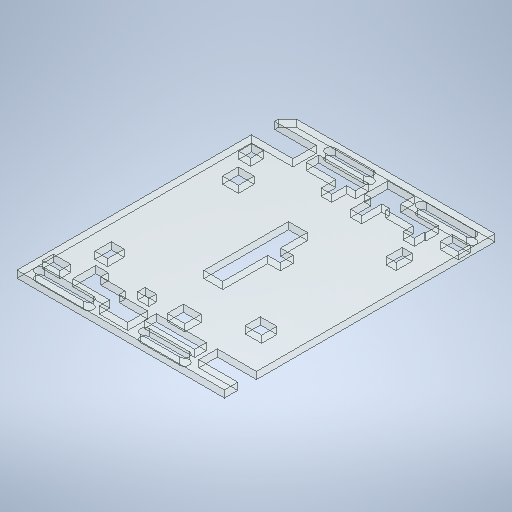
# Autodesk Inventor part: Flex Holder V1
Saved by Autodesk Inventor 2025 (Build 290162000, 162)
## iProperties
Created: 2025-07-01
Part Number: Flex Holder V1
Material: Thermoplastic Resin
Document SubType Name: Modeling
Designer: Caleb Fangmeier
Density: 1.28 g/cm^3
Appearance: Clear
Author: Caleb Fangmeier
Autodesk Inventor part; units mm, degrees
ref_plane "YZ Plane" through (0, 0, 0) normal (1, 0, 0) x (0, 1, 0)
ref_plane "XZ Plane" through (0, 0, 0) normal (0, 1, 0) x (-1, 0, 0)
ref_plane "XY Plane" through (0, 0, 0) normal (0, 0, 1) x (1, 0, 0)
sketch "Sketch1" plane through (0, 0, 0) normal (0, 1, 0) x (-1, 0, 0)
  line L0 (-22.05, -28.75) -> (22.05, -28.75)
  line L1 (22.05, -28.75) -> (22.05, 28.75)
  line L2 (22.05, 28.75) -> (-22.05, 28.75)
  line L3 (-22.05, 28.75) -> (-22.05, -28.75)
  line L4 (-22.05, -28.75) -> (22.05, 28.75) construction
  line L5 (22.05, -28.75) -> (-22.05, 28.75) construction
  point P0 (0, 0)
  dimension "d0" = 57.5
  dimension "d1" = 44.1
  constraints: 12 end point, 2 midpoint, 2 parallel, 1 horizontal, 1 perpendicular
  measures "d0" distance of L0.end L1.end
  measures "d1" distance of L1.end L2.end
extrude "Extrusion1" add sketch "Sketch1" along normal blind 1.5
sketch "Sketch4" plane through (0, 1.5, 0) normal (0, 1, 0) x (1, 0, 0)
  line L0 (22.6381, -25.9185) -> (13.7388, -25.9185)
  line L1 (13.7388, -25.9185) -> (13.7388, -21.956)
  line L2 (13.7388, -21.956) -> (22.6381, -21.956)
  line L3 (22.6381, -21.956) -> (22.6381, -25.9185)
  line L4 (11.4165, -21.956) -> (0.7633, -21.956)
  line L5 (0.7633, -21.956) -> (0.7633, -24.4569)
  line L6 (0.7633, -24.4569) -> (11.4165, -24.4569)
  line L7 (11.4165, -24.4569) -> (11.4165, -21.956)
  line L8 (-0.6658, -26.6006) -> (-6.707, -26.6006)
  line L9 (-6.707, -26.6006) -> (-6.707, -22.3783)
  line L10 (-6.707, -22.3783) -> (-0.6658, -22.3783)
  line L11 (-0.6658, -22.3783) -> (-0.6658, -26.6006)
  line L12 (-6.707, -24.392) -> (-14.5426, -24.392)
  line L13 (-14.5426, -24.392) -> (-14.5426, -21.0953)
  line L14 (-14.5426, -21.0953) -> (-6.707, -21.0953)
  line L15 (-6.707, -21.0953) -> (-6.707, -24.392)
  line L16 (-14.5426, -21.0953) -> (-11.8996, -21.0953)
  line L17 (-11.8996, -21.0953) -> (-11.8996, -19.5363)
  line L18 (-11.8996, -19.5363) -> (-14.5426, -19.5363)
  line L19 (-14.5426, -19.5363) -> (-14.5426, -21.0953)
  line L20 (-21.1238, -24.2621) -> (-17.4211, -24.2621)
  line L21 (-17.4211, -24.2621) -> (-17.4211, -21.956)
  line L22 (-17.4211, -21.956) -> (-21.1238, -21.956)
  line L23 (-21.1238, -21.956) -> (-21.1238, -24.2621)
  line L24 (5.6616, -20.7705) -> (1.894, -20.7705)
  line L25 (1.894, -20.7705) -> (1.894, -17.3277)
  line L26 (1.894, -17.3277) -> (5.6616, -17.3277)
  line L27 (5.6616, -17.3277) -> (5.6616, -20.7705)
  line L28 (-2.848, -19.9261) -> (-5.2515, -19.9261)
  line L29 (-5.2515, -19.9261) -> (-5.2515, -18.3346)
  line L30 (-5.2515, -18.3346) -> (-2.848, -18.3346)
  line L31 (-2.848, -18.3346) -> (-2.848, -19.9261)
  line L32 (-17.2689, -17.0029) -> (-14.5426, -17.0029)
  line L33 (-14.5426, -17.0029) -> (-14.5426, -13.4952)
  line L34 (-14.5426, -13.4952) -> (-17.2689, -13.4952)
  line L35 (-17.2689, -13.4952) -> (-17.2689, -17.0029)
  line L36 (15.925, -11.4814) -> (12.4173, -11.4814)
  line L37 (12.4173, -11.4814) -> (12.4173, -14.7294)
  line L38 (12.4173, -14.7294) -> (15.925, -14.7294)
  line L39 (15.925, -14.7294) -> (15.925, -11.4814)
  line L40 (-2.1335, 9.0455) -> (1.894, 9.0455)
  line L41 (1.894, 9.0455) -> (1.894, -8.9481)
  line L42 (1.894, -8.9481) -> (-2.1335, -8.9481)
  line L43 (-2.1335, -8.9481) -> (-2.1335, 9.0455)
  line L44 (4.5573, 3.3291) -> (1.6991, 3.3291)
  line L45 (1.6991, 3.3291) -> (1.6991, 0.6009)
  line L46 (1.6991, 0.6009) -> (4.5573, 0.6009)
  line L47 (4.5573, 0.6009) -> (4.5573, 3.3291)
  line L48 (-17.5287, 13.7631) -> (-14.1519, 13.7631)
  line L49 (-14.1519, 13.7631) -> (-14.1519, 10.4096)
  line L50 (-14.1519, 10.4096) -> (-17.5287, 10.4096)
  line L51 (-17.5287, 10.4096) -> (-17.5287, 13.7631)
  line L52 (16.8052, 16.3739) -> (14.7212, 16.3739)
  line L53 (14.7212, 16.3739) -> (14.7212, 12.9633)
  line L54 (14.7212, 12.9633) -> (16.8052, 12.9633)
  line L55 (16.8052, 12.9633) -> (16.8052, 16.3739)
  line L56 (-23.3919, 26.0219) -> (-13.2211, 26.0219)
  line L57 (-13.2211, 26.0219) -> (-13.2211, 21.0711)
  line L58 (-13.2211, 21.0711) -> (-23.3919, 21.0711)
  line L59 (-23.3919, 21.0711) -> (-23.3919, 26.0219)
  line L60 (-20.3793, 16.7032) -> (-17.8455, 16.7032)
  line L61 (-17.8455, 16.7032) -> (-17.8455, 19.4346)
  line L62 (-17.8455, 19.4346) -> (-20.3793, 19.4346)
  line L63 (-20.3793, 19.4346) -> (-20.3793, 16.7032)
  line L64 (-11.1745, 21.8169) -> (-0.7032, 21.8169)
  line L65 (-0.7032, 21.8169) -> (-0.7032, 24.5446)
  line L66 (-0.7032, 24.5446) -> (-11.1745, 24.5446)
  line L67 (-11.1745, 24.5446) -> (-11.1745, 21.8169)
  line L68 (-2.5673, 18.6812) -> (-4.8458, 18.6812)
  line L69 (-4.8458, 18.6812) -> (-4.8458, 22.2038)
  line L70 (-4.8458, 22.2038) -> (-2.5673, 22.2038)
  line L71 (-2.5673, 22.2038) -> (-2.5673, 18.6812)
  line L72 (0.9146, 27.1153) -> (6.539, 27.1153)
  line L73 (6.539, 27.1153) -> (6.539, 22.2038)
  line L74 (6.539, 22.2038) -> (0.9146, 22.2038)
  line L75 (0.9146, 22.2038) -> (0.9146, 27.1153)
  line L76 (2.2307, 17.9158) -> (4.5573, 17.9158)
  line L77 (4.5573, 17.9158) -> (4.5573, 22.2038)
  line L78 (4.5573, 22.2038) -> (2.2307, 22.2038)
  line L79 (2.2307, 22.2038) -> (2.2307, 17.9158)
  line L80 (6.0899, 24.1958) -> (14.5454, 24.1958)
  line L81 (14.5454, 24.1958) -> (14.5454, 21.5323)
  line L82 (14.5454, 21.5323) -> (6.0899, 21.5323)
  line L83 (6.0899, 21.5323) -> (6.0899, 24.1958)
  line L84 (14.2886, 21.5323) -> (11.9019, 21.5323)
  line L85 (11.9019, 21.5323) -> (11.9019, 19.3557)
  line L86 (11.9019, 19.3557) -> (14.2886, 19.3557)
  line L87 (14.2886, 19.3557) -> (14.2886, 21.5323)
  line L88 (21.4363, 24.0758) -> (17.64, 24.0758)
  line L89 (17.64, 24.0758) -> (17.64, 21.5323)
  line L90 (17.64, 21.5323) -> (21.4363, 21.5323)
  line L91 (21.4363, 21.5323) -> (21.4363, 24.0758)
  point P0 (0, 0)
  point P1 (6.539, 24.1958)
  point P2 (6.0899, 22.2038)
  constraints: 184 end point, 46 parallel, 23 perpendicular, 22 horizontal, 3 point on line
extrude "Clearance Cutouts" cut sketch "Sketch4" against normal blind 1.5
sketch "Sketch5" plane through (0, 1.5, 0) normal (0, 1, 0) x (1, 0, 0)
  line L0 (19.55, 26.1958) -> (9.039, 26.1958) construction
  line L1 (19.55, 27.1958) -> (9.039, 27.1958)
  line L2 (9.039, 25.1958) -> (19.55, 25.1958)
  arc A0 (19.55, 25.1958) -> (19.55, 27.1958) centre (19.55, 26.1958) ccw
  arc A1 (9.039, 27.1958) -> (9.039, 25.1958) centre (9.039, 26.1958) ccw
  line L3 (6.539, 24.1958) -> (14.5454, 24.1958) projected
  line L4 (6.539, 27.1153) -> (6.539, 24.1958) projected
  line L5 (22.05, -21.956) -> (22.05, 28.75) projected
  line L6 (-2.5854, 26.5446) -> (-10.7211, 26.5446) construction
  line L7 (-2.5854, 25.5446) -> (-10.7211, 25.5446)
  line L8 (-10.7211, 27.5446) -> (-2.5854, 27.5446)
  arc A2 (-2.5854, 25.5446) -> (-2.5854, 27.5446) centre (-2.5854, 26.5446) ccw
  arc A3 (-10.7211, 27.5446) -> (-10.7211, 25.5446) centre (-10.7211, 26.5446) ccw
  line L9 (-11.1745, 24.5446) -> (-0.7032, 24.5446) projected
  line L10 (0.9146, 22.2038) -> (0.9146, 27.1153) projected
  line L11 (-13.2211, 26.0219) -> (-13.2211, 21.0711) projected
  line L12 (-19.55, -26.392) -> (-9.207, -26.392) construction
  line L13 (-22.05, -28.75) -> (22.05, -28.75) projected
  line L14 (-19.55, -27.392) -> (-9.207, -27.392)
  line L15 (-9.207, -25.392) -> (-19.55, -25.392)
  arc A4 (-19.55, -25.392) -> (-19.55, -27.392) centre (-19.55, -26.392) ccw
  arc A5 (-9.207, -27.392) -> (-9.207, -25.392) centre (-9.207, -26.392) ccw
  line L16 (-6.707, -24.392) -> (-14.5426, -24.392) projected
  line L17 (-6.707, -26.6006) -> (-6.707, -24.392) projected
  line L18 (-22.05, 21.0711) -> (-22.05, -28.75) projected
  line L19 (2.8342, -26.4569) -> (11.2388, -26.4569) construction
  line L20 (2.8342, -27.4569) -> (11.2388, -27.4569)
  line L21 (11.2388, -25.4569) -> (2.8342, -25.4569)
  arc A6 (2.8342, -25.4569) -> (2.8342, -27.4569) centre (2.8342, -26.4569) ccw
  arc A7 (11.2388, -27.4569) -> (11.2388, -25.4569) centre (11.2388, -26.4569) ccw
  line L22 (11.4165, -24.4569) -> (0.7633, -24.4569) projected
  line L23 (-0.6658, -22.3783) -> (-0.6658, -26.6006) projected
  line L24 (13.7388, -25.9185) -> (13.7388, -21.956) projected
  point P0 (0, 0)
  point P1 (14.2945, 26.1958)
  point P2 (8.039, 26.1958)
  point P3 (20.55, 26.1958)
  point P4 (-6.6533, 26.5446)
  point P5 (-1.5854, 26.5446)
  point P6 (-11.7211, 26.5446)
  point P7 (-14.3785, -26.392)
  point P8 (-8.207, -26.392)
  point P9 (-20.55, -26.392)
  point P10 (7.0365, -26.4569)
  point P11 (1.8342, -26.4569)
  point P12 (12.2388, -26.4569)
  dimension "d23" = 2
  dimension "d24" = 1
  dimension "d25" = 1.5
  dimension "d26" = 1.5
  dimension "d27" = 1
  dimension "d28" = 2.5
  dimension "d29" = 1.5
  dimension "d30" = 1
  dimension "d31" = 1
  dimension "d32" = 1
  dimension "d33" = 1.5
  dimension "d34" = 1.5
  dimension "d35" = 1
  dimension "d36" = 1
  dimension "d37" = 2.5
  dimension "d38" = 1.5
  constraints: 32 end point, 24 point on circle, 16 tangent, 8 centre point, 5 parallel, 4 midpoint, 3 horizontal
  measures "d23" diameter of A1
  measures "d24" distance between parallel lines of L2 L3
  measures "d25" distance from line of L4 point (8.039, 26.196)
  measures "d26" distance from line of L5 point (20.55, 26.196)
  measures "d27" distance between parallel lines of L7 L9
  measures "d28" distance from line of L10 point (-1.585, 26.545)
  measures "d29" distance from line of L11 point (-11.721, 26.545)
  measures "d30" radius of A2
  measures "d31" radius of A5
  measures "d32" distance between parallel lines of L16 L15
  measures "d33" distance from line of L17 point (-8.207, -26.392)
  measures "d34" distance from line of L18 point (-20.55, -26.392)
  measures "d35" radius of A7
  measures "d36" distance between parallel lines of L22 L21
  measures "d37" distance from line of L23 point (1.834, -26.457)
  measures "d38" distance from line of L24 point (12.239, -26.457)
extrude "Extrusion4" cut sketch "Sketch5" against normal blind 1.5
chamfer "Chamfer1" distance 2 angle 45 1 edges at (-22.05, 0.75, -28.75)
body "Solid1"
